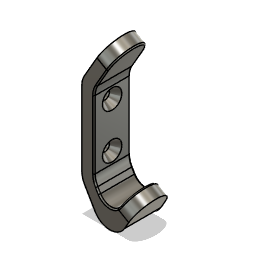
_Coat Hook.80e45464-1aeb-45e0-a7aa-d7af2d9fd1fd (Autodesk Fusion 360 design; units mm, degrees)
part number: 2025-06-09-20-10-25-206
Autodesk Fusion 360 part; units mm, degrees
sketch "Sketch1" plane through (0, 0, 0) normal (0, 0, 1) x (1, 0, 0)
  line L0 (10, 52.3205) -> (0, 35)
  line L1 (0, 35) -> (0, 0)
  line L2 (0, 0) -> (5.4848, -9.5)
  line L3 (17.6092, -9.5) -> (23.094, 0)
  line L4 (14.3301, 49.8205) -> (5, 33.6603)
  line L5 (5, 33.6603) -> (5, 1.3397)
  line L6 (5, 1.3397) -> (7.2169, -2.5)
  line L7 (15.8771, -2.5) -> (18.7639, 2.5)
  line L8 (23.094, 0) -> (18.7639, 2.5)
  line L9 (14.3301, 49.8205) -> (10, 52.3205)
  arc A0 (7.2169, -2.5) -> (15.8771, -2.5) centre (11.547, 0) ccw
  arc A1 (5.4848, -9.5) -> (17.6092, -9.5) centre (11.547, -6) ccw
  point P0 (11.547, -20)
  dimension "d1" = 35
  dimension "d2" = 20
  dimension "d3" = 20
  dimension "d4" = 20
  dimension "d5" = 150
  dimension "d6" = 150
  dimension "d8" = 5
  dimension "d9" = 7
  constraint coincident L1.end L2.start
  constraint vertical L1
  constraint parallel L0 L3
  constraint perpendicular L0 L9
  constraint tangent L6 A0
  constraint tangent L7 A0
  constraint coincident P0 L2
  constraint coincident P0 L3
  constraint tangent L2 A1
  constraint tangent L3 A1
  measures "d1" distance of L0.end L1.end
  measures "d2" distance of L0.start L0.end
  measures "d3" vertical distance of L1.end P0
  measures "d4" vertical distance of P0 L3.end
  measures "d5" angle of L0 L1
  measures "d6" angle of L1 L2
  measures "d8" radius of A0
  measures "d9" radius of A1
extrude "Extrude1" add sketch "Sketch1" along normal blind 15
sketch "Sketch2" plane through (5, 0, 0) normal (1, 0, 0) x (0, 0, -1)
  line L0 (0, 1.3397) -> (0, 33.6603)
  line L1 (0, 33.6603) -> (-15, 33.6603)
  line L2 (-15, 33.6603) -> (-15, 1.3397)
  line L3 (-15, 1.3397) -> (0, 1.3397)
  line L4 (-7.5, 1.3397) -> (-7.5, 33.6603) construction
  line L5 (-15, 17.5) -> (0, 17.5) construction
  circle A0 centre (-7.5, 26.7565) radius 4
  circle A1 centre (-7.5, 8.2435) radius 4
  dimension "d12" = 8
  dimension "d13" = 6.9037
  constraint midpoint L3 L4.start
  constraint midpoint L1 L4.end
  constraint midpoint L2 L5.start
  constraint midpoint L0 L5.end
  constraint coincident L4 A0.centre
  constraint symmetric L5 A0 A1
  measures "d12" diameter of A0
  measures "d13" distance of L4.end A0.centre
extrude "Extrude2" cut sketch "Sketch2" against normal blind 3 draft -35 contours A0 | A1
extrude "Extrude3" cut 2 faces at (2, 27.3459, 7.7313) (2, 8.7385, 7.1999) along direction (-1, 0, 0) through all
fillet "Fillet1" radius 7.5 4 edges at (20.9289, 1.25, 15) (20.9289, 1.25, 0) (12.1651, 51.0705, 15) (12.1651, 51.0705, 0)
fillet "Fillet2" radius 8 4 edges at (5, 1.3397, 7.5) (0, 0, 7.5) (0, 35, 7.5) (5, 33.6603, 7.5)
fillet "Fillet3" radius 0.5 16 edges at (5.2726, 33.5872, 15) (8.326, 39.421, 15) (14.3301, 49.8205, 7.5) (8.326, 39.421, 0) (5.2726, 33.5872, 0) (5, 17.5, 0) (5.2726, 1.4128, 0) (6.6443, -1.5083, 0) (10.6702, -4.9225, 0) (15.3815, -3.2072, 0.0512) (18.7639, 2.5, 7.5) (15.3815, -3.2072, 14.9488) (10.6702, -4.9225, 15) (6.6443, -1.5083, 15) (5.2726, 1.4128, 15) (5, 17.5, 15)
equation "d3 = d2"
equation "d4 = d2"
equation "d6 = d5"
